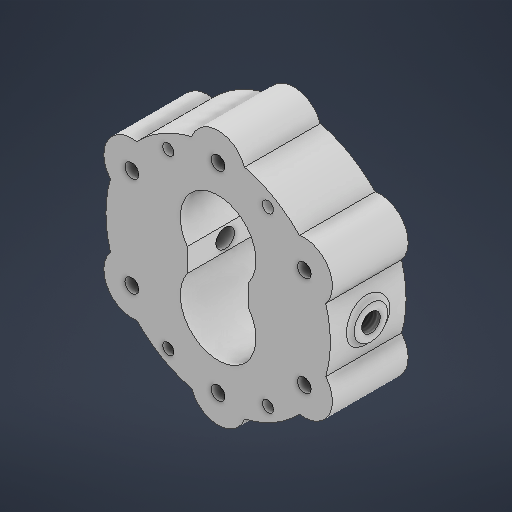
# Autodesk Inventor part: B1
Saved by Autodesk Inventor 2025.4 (Build 294407000, 407)
## iProperties
Created: 2026-05-18
Part Number: B1
Material: Generic
Document SubType Name: Modeling
Designer: VuQuan
Density: 1 g/cm^3
Appearance: Default
Author: VuQuan
Autodesk Inventor part; units mm, degrees
note: some values were not read from the file. Chosen so that the rebuilt part matches the saved one: direction of "Hole2".
ref_plane "XZ Plane" through (0, 0, 0) normal (0, 1, 0) x (-1, 0, 0)
sketch "Sketch1" plane through (0, 0, 0) normal (0, 0, 1) x (1, 0, 0)
  circle A0 centre (0, 0) radius 35.5 construction
  circle A1 centre (17.75, 30.7439) radius 2
  line L0 (17.75, 30.7439) -> (0, 0) construction
  line L1 (0, 35.5) -> (0, -35.5) construction
  line L2 (35.5, 0) -> (-35.5, 0) construction
  circle A2 centre (-17.75, 30.7439) radius 2
  circle A3 centre (17.75, -30.7439) radius 2
  circle A4 centre (-17.75, -30.7439) radius 2
  line L3 (-11, 4.1738) -> (-11, 0)
  line L4 (11, 0) -> (11, 4.1738)
  arc A5 (11, 4.1738) -> (-11, 4.1738) centre (0, 12) ccw
  line L5 (-11, -4.1738) -> (-11, 0)
  line L6 (11, 0) -> (11, -4.1738)
  arc A6 (-11, -4.1738) -> (11, -4.1738) centre (0, -12) ccw
  arc A7 (28.962, 27.59) -> (9.4126, 38.8768) centre (0, 0) ccw
  arc A8 (9.4126, 38.8768) -> (-9.4126, 38.8768) centre (0, 35.5) ccw
  arc A9 (-28.962, 27.59) -> (-38.3746, 11.2868) centre (-30.7439, 17.75) ccw
  arc A10 (-9.4126, 38.8768) -> (-28.962, 27.59) centre (0, 0) ccw
  arc A11 (-38.3746, -11.2868) -> (-28.962, -27.59) centre (-30.7439, -17.75) ccw
  arc A12 (-38.3746, 11.2868) -> (-38.3746, -11.2868) centre (0, 0) ccw
  arc A13 (-9.4126, -38.8768) -> (9.4126, -38.8768) centre (0, -35.5) ccw
  arc A14 (-28.962, -27.59) -> (-9.4126, -38.8768) centre (0, 0) ccw
  arc A15 (28.962, -27.59) -> (38.3746, -11.2868) centre (30.7439, -17.75) ccw
  arc A16 (9.4126, -38.8768) -> (28.962, -27.59) centre (0, 0) ccw
  arc A17 (38.3746, 11.2868) -> (28.962, 27.59) centre (30.7439, 17.75) ccw
  arc A18 (38.3746, -11.2868) -> (38.3746, 11.2868) centre (0, 0) ccw
  point P0 (-30.7439, 17.75)
  point P1 (-30.7439, 17.75)
  point P2 (-30.7439, -17.75)
  point P3 (-30.7439, -17.75)
  point P4 (0, -35.5)
  point P5 (0, -35.5)
  point P6 (30.7439, -17.75)
  point P7 (30.7439, -17.75)
  point P8 (30.7439, 17.75)
  point P9 (30.7439, 17.75)
  point P10 (28.962, 27.59)
  point P11 (-9.4126, 38.8768)
  point P12 (-38.3746, 11.2868)
  point P13 (-28.962, -27.59)
  point P14 (9.4126, -38.8768)
  point P15 (38.3746, -11.2868)
  dimension "d0" = 35.5
  dimension "d2" = 30
  dimension "d4" = 13.5
  dimension "d5" = 24
  dimension "d6" = 22
  dimension "d10" = 360
  dimension "d15" = 40
  dimension "d16" = 10
  dimension "d19" = 360
  dimension "d21" = 4
  constraints: 33 point on circle, 19 centre point, 14 end point, 10 coincident, 6 symmetric about line, 4 point on line, 2 midpoint, 2 vertical, 1 horizontal, 1 horizontal alignment, 1 parallel, 1 perpendicular, 60 other
  measures "d0" radius of A0
  measures "d2" angle of L1 L0
  measures "d4" radius of A5
  measures "d5" distance of A6.centre A5.centre
  measures "d6" distance between parallel lines of L4 L3
  measures "d15" radius of A7
  measures "d16" radius of A8
  measures "d21" diameter of A1
extrude "Extrusion1" add sketch "Sketch1" along normal blind 27
hole "Hole1" at (-30.7439, 17.75, 0) at (-30.7439, -17.75, 0) at (0, -35.5, 0) at (30.7439, -17.75, 0) at (30.7439, 17.75, 0) at (0, 35.5, 0) direction (0, 0, 1) diameter 4.917 end through all thread size "M6x1" class "6H" standard "ANSI Metric M Profile"
ref_plane "Work Plane1" through (41, 0, 0) normal (1, 0, 0) x (0, 1, 0)
sketch "Sketch2" plane through (41, 0, 0) normal (1, 0, 0) x (0, 1, 0)
  line L0 (-11.2868, 0) -> (11.2868, 0) projected
  line L1 (11.2868, 0) -> (11.2868, 27) projected
  line L2 (-11.2868, 27) -> (11.2868, 27) projected
  line L3 (-11.2868, 0) -> (-11.2868, 27) projected
  circle A0 centre (0, 13.5) radius 6
  point P0 (0, 0)
  point P1 (-11.2868, 13.5)
  point P2 (0, 0)
  dimension "d33" = 12
  constraints: 2 midpoint, 1 centre point, 1 horizontal alignment, 1 vertical alignment
  measures "d33" diameter of A0
extrude "Extrusion2" add sketch "Sketch2" against normal up to surface contours A0
ref_plane "Work Plane2" through (28.962, 27.59, 0) normal (1, 0, 0) x (0, 0, 1)
sketch "Sketch5" plane through (41, 0, 13.5) normal (1, 0, 0) x (0, 0, -1)
  circle A0 centre (0, 0) radius 6 projected
  point P0 (13.5, 0)
  constraints: 1 coincident
hole "Hole2" at (41, 0, 13.5) direction (-1, 0, 0) diameter 6.647 depth 30 thread size "M8x1.25" class "6H" standard "ISO Metric profile"
mirror "Mirror1" about plane through (0, 0, 0) normal (1, 0, 0) of "Extrusion2", "Hole2"
fillet "Fillet1" radius 2 2 edges at (39.5475, -5.9999, 13.4667) (-39.5475, -5.9999, 13.4667)
body "Solid1"
